Autodesk Fusion 360 part; units mm, degrees
(part 3 of 8)
  spline S11 degree 5 poles (2.5437, 23.8648) (2.5417, 23.8617) (2.5376, 23.8555) (2.5314, 23.8462) (2.5232, 23.8338) (2.5131, 23.8183) (2.503, 23.8028) (2.4929, 23.7874) (2.4829, 23.7719) (2.4729, 23.7565) (2.4629, 23.7411) (2.4531, 23.7257) (2.4432, 23.7103) (2.4334, 23.695) (2.4237, 23.6796) (2.414, 23.6643) (2.4044, 23.649) (2.3948, 23.6337) (2.3852, 23.6184) (2.3757, 23.6032) (2.3663, 23.588) (2.3569, 23.5727) (2.3475, 23.5575) (2.3382, 23.5424) (2.3289, 23.5272) (2.3197, 23.5121) (2.3105, 23.4969) (2.3014, 23.4818) (2.2923, 23.4668) (2.2833, 23.4517) (2.2743, 23.4367) (2.2654, 23.4216) (2.2565, 23.4066) (2.2477, 23.3917) (2.2389, 23.3767) (2.2302, 23.3618) (2.2215, 23.3468) (2.2128, 23.332) (2.2043, 23.3171) (2.1957, 23.3022) (2.1872, 23.2874) (2.1788, 23.2726) (2.1703, 23.2578) (2.162, 23.2431) (2.1537, 23.2283) (2.1454, 23.2136) (2.1372, 23.1989) (2.129, 23.1843) (2.1209, 23.1696) (2.1129, 23.155) (2.1048, 23.1404) (2.0969, 23.1259) (2.0889, 23.1113) (2.0811, 23.0968) (2.0732, 23.0823) (2.0654, 23.0679) (2.0577, 23.0535) (2.05, 23.039) (2.0424, 23.0247) (2.0348, 23.0103) (2.0272, 22.996) (2.0197, 22.9817) (2.0123, 22.9674) (2.0049, 22.9532) (1.9975, 22.939) (1.9902, 22.9248) (1.983, 22.9106) (1.9758, 22.8965) (1.9686, 22.8824) (1.9615, 22.8683) (1.9544, 22.8543) (1.9474, 22.8403) (1.9404, 22.8263) (1.9335, 22.8124) (1.9266, 22.7984) (1.9198, 22.7846) (1.913, 22.7707) (1.9063, 22.7569) (1.8996, 22.7431) (1.8929, 22.7293) (1.8863, 22.7156) (1.8798, 22.7019) (1.8733, 22.6883) (1.8668, 22.6747) (1.8604, 22.6611) (1.8541, 22.6475) (1.8478, 22.634) (1.8415, 22.6205) (1.8353, 22.6071) (1.8291, 22.5936) (1.823, 22.5803) (1.8169, 22.5669) (1.8109, 22.5536) (1.8049, 22.5403) (1.799, 22.5271) (1.7931, 22.5139) (1.7873, 22.5008) (1.7815, 22.4876) (1.7757, 22.4746) (1.77, 22.4615) (1.7644, 22.4485) (1.7588, 22.4356) (1.7532, 22.4226) (1.7477, 22.4097) (1.7423, 22.3969) (1.7368, 22.3841) (1.7315, 22.3713) (1.7261, 22.3586) (1.7209, 22.3459) (1.7156, 22.3333) (1.7105, 22.3207) (1.7053, 22.3082) (1.7002, 22.2956) (1.6952, 22.2832) (1.6902, 22.2708) (1.6853, 22.2584) (1.6803, 22.2461) (1.6755, 22.2338) (1.6707, 22.2215) (1.6659, 22.2093) (1.6612, 22.1972) (1.6565, 22.1851) (1.6519, 22.173) (1.6473, 22.161) (1.6428, 22.1491) (1.6383, 22.1372) (1.6339, 22.1253) (1.6295, 22.1135) (1.6251, 22.1017) (1.6208, 22.09) (1.6165, 22.0784) (1.6123, 22.0668) (1.6082, 22.0552) (1.604, 22.0437) (1.6, 22.0322) (1.5959, 22.0208) (1.592, 22.0095) (1.588, 21.9982) (1.5841, 21.987) (1.5803, 21.9758) (1.5765, 21.9646) (1.5727, 21.9536) (1.569, 21.9425) (1.5653, 21.9316) (1.5617, 21.9207) (1.5581, 21.9098) (1.5546, 21.899) (1.5511, 21.8883) (1.5476, 21.8776) (1.5442, 21.867) (1.5409, 21.8565) (1.5376, 21.846) (1.5343, 21.8356) (1.5311, 21.8252) (1.5279, 21.8149) (1.5247, 21.8047) (1.5216, 21.7945) (1.5186, 21.7844) (1.5156, 21.7743) (1.5126, 21.7644) (1.5097, 21.7544) (1.5068, 21.7446) (1.504, 21.7348) (1.5012, 21.7251) (1.4984, 21.7155) (1.4957, 21.7059) (1.4931, 21.6964) (1.4905, 21.687) (1.4879, 21.6776) (1.4853, 21.6683) (1.4828, 21.6591) (1.4804, 21.65) (1.478, 21.6409) (1.4756, 21.6319) (1.4733, 21.623) (1.471, 21.6142) (1.4688, 21.6054) (1.4666, 21.5967) (1.4644, 21.5881) (1.4623, 21.5796) (1.4602, 21.5711) (1.4582, 21.5628) (1.4562, 21.5545) (1.4542, 21.5463) (1.4523, 21.5382) (1.4504, 21.5302) (1.4486, 21.5222) (1.4468, 21.5144) (1.445, 21.5066) (1.4433, 21.4989) (1.4416, 21.4913) (1.44, 21.4838) (1.4384, 21.4764) (1.4368, 21.4691) (1.4353, 21.4619) (1.4338, 21.4548) (1.4324, 21.4478) (1.431, 21.4408) (1.4296, 21.434) (1.4283, 21.4273) (1.427, 21.4206) (1.4257, 21.4141) (1.4245, 21.4077) (1.4233, 21.4014) (1.4221, 21.3951) (1.421, 21.389) (1.4199, 21.383) (1.4189, 21.3771) (1.4179, 21.3714) (1.4169, 21.3657) (1.416, 21.3602) (1.4151, 21.3547) (1.4142, 21.3494) (1.4134, 21.3442) (1.4125, 21.3391) (1.4118, 21.3342) (1.411, 21.3293) (1.4103, 21.3246) (1.4096, 21.32) (1.409, 21.3156) (1.4084, 21.3113) (1.4078, 21.3071) (1.4072, 21.303) (1.4067, 21.2991) (1.4062, 21.2953) (1.4058, 21.2917) (1.4053, 21.2882) (1.4049, 21.2849) (1.4045, 21.2817) (1.4042, 21.2786) (1.4038, 21.2758) (1.4035, 21.273) (1.4033, 21.2705) (1.403, 21.2681) (1.4028, 21.2658) (1.4026, 21.2637) (1.4024, 21.2618) (1.4022, 21.2601) (1.4021, 21.2586) (1.402, 21.2572) (1.4019, 21.256) (1.4018, 21.2552) (1.4018, 21.2547) (1.4017, 21.2544) (1.4017, 21.2543) knots -1 -1 -1 -1 -1 -1 -0.99583333 -0.99166667 -0.9875 -0.98333333 -0.97916667 -0.975 -0.97083333 -0.96666667 -0.9625 -0.95833333 -0.95416667 -0.95 -0.94583333 -0.94166667 -0.9375 -0.93333333 -0.92916667 -0.925 -0.92083333 -0.91666667 -0.9125 -0.90833333 -0.90416667 -0.9 -0.89583333 -0.89166667 -0.8875 -0.88333333 -0.87916667 -0.875 -0.87083333 -0.86666667 -0.8625 -0.85833333 -0.85416667 -0.85 -0.84583333 -0.84166667 -0.8375 -0.83333333 -0.82916667 -0.825 -0.82083333 -0.81666667 -0.8125 -0.80833333 -0.80416667 -0.8 -0.79583333 -0.79166667 -0.7875 -0.78333333 -0.77916667 -0.775 -0.77083333 -0.76666667 -0.7625 -0.75833333 -0.75416667 -0.75 -0.74583333 -0.74166667 -0.7375 -0.73333333 -0.72916667 -0.725 -0.72083333 -0.71666667 -0.7125 -0.70833333 -0.70416667 -0.7 -0.69583333 -0.69166667 -0.6875 -0.68333333 -0.67916667 -0.675 -0.67083333 -0.66666667 -0.6625 -0.65833333 -0.65416667 -0.65 -0.64583333 -0.64166667 -0.6375 -0.63333333 -0.62916667 -0.625 -0.62083333 -0.61666667 -0.6125 -0.60833333 -0.60416667 -0.6 -0.59583333 -0.59166667 -0.5875 -0.58333333 -0.57916667 -0.575 -0.57083333 -0.56666667 -0.5625 -0.55833333 -0.55416667 -0.55 -0.54583333 -0.54166667 -0.5375 -0.53333333 -0.52916667 -0.525 -0.52083333 -0.51666667 -0.5125 -0.50833333 -0.50416667 -0.5 -0.49583333 -0.49166667 -0.4875 -0.48333333 -0.47916667 -0.475 -0.47083333 -0.46666667 -0.4625 -0.45833333 -0.45416667 -0.45 -0.44583333 -0.44166667 -0.4375 -0.43333333 -0.42916667 -0.425 -0.42083333 -0.41666667 -0.4125 -0.40833333 -0.40416667 -0.4 -0.39583333 -0.39166667 -0.3875 -0.38333333 -0.37916667 -0.375 -0.37083333 -0.36666667 -0.3625 -0.35833333 -0.35416667 -0.35 -0.34583333 -0.34166667 -0.3375 -0.33333333 -0.32916667 -0.325 -0.32083333 -0.31666667 -0.3125 -0.30833333 -0.30416667 -0.3 -0.29583333 -0.29166667 -0.2875 -0.28333333 -0.27916667 -0.275 -0.27083333 -0.26666667 -0.2625 -0.25833333 -0.25416667 -0.25 -0.24583333 -0.24166667 -0.2375 -0.23333333 -0.22916667 -0.225 -0.22083333 -0.21666667 -0.2125 -0.20833333 -0.20416667 -0.2 -0.19583333 -0.19166667 -0.1875 -0.18333333 -0.17916667 -0.175 -0.17083333 -0.16666667 -0.1625 -0.15833333 -0.15416667 -0.15 -0.14583333 -0.14166667 -0.1375 -0.13333333 -0.12916667 -0.125 -0.12083333 -0.11666667 -0.1125 -0.10833333 -0.10416667 -0.1 -0.09583333 -0.09166667 -0.0875 -0.08333333 -0.07916667 -0.075 -0.07083333 -0.06666667 -0.0625 -0.05833333 -0.05416667 -0.05 -0.04583333 -0.04166667 -0.0375 -0.03333333 -0.02916667 -0.025 -0.02083333 -0.01666667 -0.0125 -0.00833333 -0.00416667 0 0 0 0 0 0
  line L22 (1.4017, 21.2543) -> (1.4016, 21.2531)
  line L23 (1.4016, 21.2531) -> (1.2832, 19.4577)
  arc A12 (1.2832, 19.4577) -> (-1.2832, 19.4577) centre (0, 0) ccw
  line L24 (-1.2832, 19.4577) -> (-1.4016, 21.2531)
  line L25 (-1.4016, 21.2531) -> (-1.4017, 21.2543)
  spline S12 degree 5 poles (-1.4017, 21.2543) (-1.4017, 21.2544) (-1.4018, 21.2547) (-1.4018, 21.2552) (-1.4019, 21.256) (-1.402, 21.2572) (-1.4021, 21.2586) (-1.4022, 21.2601) (-1.4024, 21.2618) (-1.4026, 21.2637) (-1.4028, 21.2658) (-1.403, 21.2681) (-1.4033, 21.2705) (-1.4035, 21.273) (-1.4038, 21.2758) (-1.4042, 21.2786) (-1.4045, 21.2817) (-1.4049, 21.2849) (-1.4053, 21.2882) (-1.4058, 21.2917) (-1.4062, 21.2953) (-1.4067, 21.2991) (-1.4072, 21.303) (-1.4078, 21.3071) (-1.4084, 21.3113) (-1.409, 21.3156) (-1.4096, 21.32) (-1.4103, 21.3246) (-1.411, 21.3293) (-1.4118, 21.3342) (-1.4125, 21.3391) (-1.4134, 21.3442) (-1.4142, 21.3494) (-1.4151, 21.3547) (-1.416, 21.3602) (-1.4169, 21.3657) (-1.4179, 21.3714) (-1.4189, 21.3771) (-1.4199, 21.383) (-1.421, 21.389) (-1.4221, 21.3951) (-1.4233, 21.4014) (-1.4245, 21.4077) (-1.4257, 21.4141) (-1.427, 21.4206) (-1.4283, 21.4273) (-1.4296, 21.434) (-1.431, 21.4408) (-1.4324, 21.4478) (-1.4338, 21.4548) (-1.4353, 21.4619) (-1.4368, 21.4691) (-1.4384, 21.4764) (-1.44, 21.4838) (-1.4416, 21.4913) (-1.4433, 21.4989) (-1.445, 21.5066) (-1.4468, 21.5144) (-1.4486, 21.5222) (-1.4504, 21.5302) (-1.4523, 21.5382) (-1.4542, 21.5463) (-1.4562, 21.5545) (-1.4582, 21.5628) (-1.4602, 21.5711) (-1.4623, 21.5796) (-1.4644, 21.5881) (-1.4666, 21.5967) (-1.4688, 21.6054) (-1.471, 21.6142) (-1.4733, 21.623) (-1.4756, 21.6319) (-1.478, 21.6409) (-1.4804, 21.65) (-1.4828, 21.6591) (-1.4853, 21.6683) (-1.4879, 21.6776) (-1.4905, 21.687) (-1.4931, 21.6964) (-1.4957, 21.7059) (-1.4984, 21.7155) (-1.5012, 21.7251) (-1.504, 21.7348) (-1.5068, 21.7446) (-1.5097, 21.7544) (-1.5126, 21.7644) (-1.5156, 21.7743) (-1.5186, 21.7844) (-1.5216, 21.7945) (-1.5247, 21.8047) (-1.5279, 21.8149) (-1.5311, 21.8252) (-1.5343, 21.8356) (-1.5376, 21.846) (-1.5409, 21.8565) (-1.5442, 21.867) (-1.5476, 21.8776) (-1.5511, 21.8883) (-1.5546, 21.899) (-1.5581, 21.9098) (-1.5617, 21.9207) (-1.5653, 21.9316) (-1.569, 21.9425) (-1.5727, 21.9536) (-1.5765, 21.9646) (-1.5803, 21.9758) (-1.5841, 21.987) (-1.588, 21.9982) (-1.592, 22.0095) (-1.5959, 22.0208) (-1.6, 22.0322) (-1.604, 22.0437) (-1.6082, 22.0552) (-1.6123, 22.0668) (-1.6165, 22.0784) (-1.6208, 22.09) (-1.6251, 22.1017) (-1.6295, 22.1135) (-1.6339, 22.1253) (-1.6383, 22.1372) (-1.6428, 22.1491) (-1.6473, 22.161) (-1.6519, 22.173) (-1.6565, 22.1851) (-1.6612, 22.1972) (-1.6659, 22.2093) (-1.6707, 22.2215) (-1.6755, 22.2338) (-1.6803, 22.2461) (-1.6853, 22.2584) (-1.6902, 22.2708) (-1.6952, 22.2832) (-1.7002, 22.2956) (-1.7053, 22.3082) (-1.7105, 22.3207) (-1.7156, 22.3333) (-1.7209, 22.3459) (-1.7261, 22.3586) (-1.7315, 22.3713) (-1.7368, 22.3841) (-1.7423, 22.3969) (-1.7477, 22.4097) (-1.7532, 22.4226) (-1.7588, 22.4356) (-1.7644, 22.4485) (-1.77, 22.4615) (-1.7757, 22.4746) (-1.7815, 22.4876) (-1.7873, 22.5008) (-1.7931, 22.5139) (-1.799, 22.5271) (-1.8049, 22.5403) (-1.8109, 22.5536) (-1.8169, 22.5669) (-1.823, 22.5803) (-1.8291, 22.5936) (-1.8353, 22.6071) (-1.8415, 22.6205) (-1.8478, 22.634) (-1.8541, 22.6475) (-1.8604, 22.6611) (-1.8668, 22.6747) (-1.8733, 22.6883) (-1.8798, 22.7019) (-1.8863, 22.7156) (-1.8929, 22.7293) (-1.8996, 22.7431) (-1.9063, 22.7569) (-1.913, 22.7707) (-1.9198, 22.7846) (-1.9266, 22.7984) (-1.9335, 22.8124) (-1.9404, 22.8263) (-1.9474, 22.8403) (-1.9544, 22.8543) (-1.9615, 22.8683) (-1.9686, 22.8824) (-1.9758, 22.8965) (-1.983, 22.9106) (-1.9902, 22.9248) (-1.9975, 22.939) (-2.0049, 22.9532) (-2.0123, 22.9674) (-2.0197, 22.9817) (-2.0272, 22.996) (-2.0348, 23.0103) (-2.0424, 23.0247) (-2.05, 23.039) (-2.0577, 23.0535) (-2.0654, 23.0679) (-2.0732, 23.0823) (-2.0811, 23.0968) (-2.0889, 23.1113) (-2.0969, 23.1259) (-2.1048, 23.1404) (-2.1129, 23.155) (-2.1209, 23.1696) (-2.129, 23.1843) (-2.1372, 23.1989) (-2.1454, 23.2136) (-2.1537, 23.2283) (-2.162, 23.2431) (-2.1703, 23.2578) (-2.1788, 23.2726) (-2.1872, 23.2874) (-2.1957, 23.3022) (-2.2043, 23.3171) (-2.2128, 23.332) (-2.2215, 23.3468) (-2.2302, 23.3618) (-2.2389, 23.3767) (-2.2477, 23.3917) (-2.2565, 23.4066) (-2.2654, 23.4216) (-2.2743, 23.4367) (-2.2833, 23.4517) (-2.2923, 23.4668) (-2.3014, 23.4818) (-2.3105, 23.4969) (-2.3197, 23.5121) (-2.3289, 23.5272) (-2.3382, 23.5424) (-2.3475, 23.5575) (-2.3569, 23.5727) (-2.3663, 23.588) (-2.3757, 23.6032) (-2.3852, 23.6184) (-2.3948, 23.6337) (-2.4044, 23.649) (-2.414, 23.6643) (-2.4237, 23.6796) (-2.4334, 23.695) (-2.4432, 23.7103) (-2.4531, 23.7257) (-2.4629, 23.7411) (-2.4729, 23.7565) (-2.4829, 23.7719) (-2.4929, 23.7874) (-2.503, 23.8028) (-2.5131, 23.8183) (-2.5232, 23.8338) (-2.5314, 23.8462) (-2.5376, 23.8555) (-2.5417, 23.8617) (-2.5437, 23.8648) knots 0 0 0 0 0 0 0.00416667 0.00833333 0.0125 0.01666667 0.02083333 0.025 0.02916667 0.03333333 0.0375 0.04166667 0.04583333 0.05 0.05416667 0.05833333 0.0625 0.06666667 0.07083333 0.075 0.07916667 0.08333333 0.0875 0.09166667 0.09583333 0.1 0.10416667 0.10833333 0.1125 0.11666667 0.12083333 0.125 0.12916667 0.13333333 0.1375 0.14166667 0.14583333 0.15 0.15416667 0.15833333 0.1625 0.16666667 0.17083333 0.175 0.17916667 0.18333333 0.1875 0.19166667 0.19583333 0.2 0.20416667 0.20833333 0.2125 0.21666667 0.22083333 0.225 0.22916667 0.23333333 0.2375 0.24166667 0.24583333 0.25 0.25416667 0.25833333 0.2625 0.26666667 0.27083333 0.275 0.27916667 0.28333333 0.2875 0.29166667 0.29583333 0.3 0.30416667 0.30833333 0.3125 0.31666667 0.32083333 0.325 0.32916667 0.33333333 0.3375 0.34166667 0.34583333 0.35 0.35416667 0.35833333 0.3625 0.36666667 0.37083333 0.375 0.37916667 0.38333333 0.3875 0.39166667 0.39583333 0.4 0.40416667 0.40833333 0.4125 0.41666667 0.42083333 0.425 0.42916667 0.43333333 0.4375 0.44166667 0.44583333 0.45 0.45416667 0.45833333 0.4625 0.46666667 0.47083333 0.475 0.47916667 0.48333333 0.4875 0.49166667 0.49583333 0.5 0.50416667 0.50833333 0.5125 0.51666667 0.52083333 0.525 0.52916667 0.53333333 0.5375 0.54166667 0.54583333 0.55 0.55416667 0.55833333 0.5625 0.56666667 0.57083333 0.575 0.57916667 0.58333333 0.5875 0.59166667 0.59583333 0.6 0.60416667 0.60833333 0.6125 0.61666667 0.62083333 0.625 0.62916667 0.63333333 0.6375 0.64166667 0.64583333 0.65 0.65416667 0.65833333 0.6625 0.66666667 0.67083333 0.675 0.67916667 0.68333333 0.6875 0.69166667 0.69583333 0.7 0.70416667 0.70833333 0.7125 0.71666667 0.72083333 0.725 0.72916667 0.73333333 0.7375 0.74166667 0.74583333 0.75 0.75416667 0.75833333 0.7625 0.76666667 0.77083333 0.775 0.77916667 0.78333333 0.7875 0.79166667 0.79583333 0.8 0.80416667 0.80833333 0.8125 0.81666667 0.82083333 0.825 0.82916667 0.83333333 0.8375 0.84166667 0.84583333 0.85 0.85416667 0.85833333 0.8625 0.86666667 0.87083333 0.875 0.87916667 0.88333333 0.8875 0.89166667 0.89583333 0.9 0.90416667 0.90833333 0.9125 0.91666667 0.92083333 0.925 0.92916667 0.93333333 0.9375 0.94166667 0.94583333 0.95 0.95416667 0.95833333 0.9625 0.96666667 0.97083333 0.975 0.97916667 0.98333333 0.9875 0.99166667 0.99583333 1 1 1 1 1 1
  arc A13 (-2.5437, 23.8648) -> (-4.2828, 23.6148) centre (0, 0) ccw
  spline S13 degree 5 poles (-4.2828, 23.6148) (-4.2839, 23.6112) (-4.2861, 23.6041) (-4.2894, 23.5934) (-4.2937, 23.5792) (-4.2991, 23.5615) (-4.3045, 23.5438) (-4.3098, 23.5261) (-4.315, 23.5085) (-4.3203, 23.4909) (-4.3255, 23.4733) (-4.3306, 23.4558) (-4.3357, 23.4382) (-4.3408, 23.4207) (-4.3458, 23.4033) (-4.3508, 23.3858) (-4.3557, 23.3684) (-4.3606, 23.3511) (-4.3655, 23.3337) (-4.3703, 23.3164) (-4.3751, 23.2991) (-4.3798, 23.2819) (-4.3845, 23.2647) (-4.3892, 23.2475) (-4.3938, 23.2303) (-4.3984, 23.2132) (-4.4029, 23.1961) (-4.4074, 23.179) (-4.4119, 23.162) (-4.4163, 23.145) (-4.4206, 23.1281) (-4.425, 23.1111) (-4.4293, 23.0942) (-4.4335, 23.0774) (-4.4378, 23.0606) (-4.4419, 23.0438) (-4.4461, 23.027) (-4.4502, 23.0103) (-4.4542, 22.9936) (-4.4582, 22.9769) (-4.4622, 22.9603) (-4.4662, 22.9437) (-4.4701, 22.9272) (-4.4739, 22.9107) (-4.4777, 22.8942) (-4.4815, 22.8777) (-4.4853, 22.8613) (-4.489, 22.845) (-4.4926, 22.8286) (-4.4963, 22.8124) (-4.4998, 22.7961) (-4.5034, 22.7799) (-4.5069, 22.7637) (-4.5104, 22.7475) (-4.5138, 22.7314) (-4.5172, 22.7154) (-4.5206, 22.6993) (-4.5239, 22.6834) (-4.5272, 22.6674) (-4.5304, 22.6515) (-4.5336, 22.6356) (-4.5368, 22.6198) (-4.5399, 22.604) (-4.543, 22.5883) (-4.546, 22.5725) (-4.549, 22.5569) (-4.552, 22.5412) (-4.555, 22.5257) (-4.5579, 22.5101) (-4.5607, 22.4946) (-4.5636, 22.4792) (-4.5663, 22.4637) (-4.5691, 22.4484) (-4.5718, 22.433) (-4.5745, 22.4177) (-4.5771, 22.4025) (-4.5797, 22.3873) (-4.5823, 22.3721) (-4.5848, 22.357) (-4.5873, 22.3419) (-4.5898, 22.3269) (-4.5922, 22.3119) (-4.5946, 22.297) (-4.597, 22.2821) (-4.5993, 22.2673) (-4.6016, 22.2525) (-4.6038, 22.2377) (-4.606, 22.223) (-4.6082, 22.2084) (-4.6103, 22.1938) (-4.6124, 22.1792) (-4.6145, 22.1647) (-4.6165, 22.1502) (-4.6185, 22.1358) (-4.6205, 22.1214) (-4.6224, 22.1071) (-4.6243, 22.0929) (-4.6262, 22.0786) (-4.628, 22.0645) (-4.6298, 22.0503) (-4.6316, 22.0363) (-4.6333, 22.0223) (-4.635, 22.0083) (-4.6366, 21.9944) (-4.6383, 21.9805) (-4.6398, 21.9667) (-4.6414, 21.953) (-4.6429, 21.9392) (-4.6444, 21.9256) (-4.6459, 21.912) (-4.6473, 21.8985) (-4.6487, 21.885) (-4.65, 21.8715) (-4.6514, 21.8582) (-4.6527, 21.8448) (-4.6539, 21.8316) (-4.6552, 21.8183) (-4.6564, 21.8052) (-4.6575, 21.7921) (-4.6587, 21.779) (-4.6598, 21.7661) (-4.6608, 21.7531) (-4.6619, 21.7403) (-4.6629, 21.7275) (-4.6639, 21.7147) (-4.6648, 21.702) (-4.6657, 21.6894) (-4.6666, 21.6768) (-4.6675, 21.6643) (-4.6683, 21.6519) (-4.6691, 21.6395) (-4.6699, 21.6271) (-4.6706, 21.6149) (-4.6714, 21.6027) (-4.672, 21.5905) (-4.6727, 21.5785) (-4.6733, 21.5664) (-4.6739, 21.5545) (-4.6745, 21.5426) (-4.675, 21.5308) (-4.6756, 21.5191) (-4.676, 21.5074) (-4.6765, 21.4958) (-4.6769, 21.4842) (-4.6773, 21.4727) (-4.6777, 21.4613) (-4.6781, 21.45) (-4.6784, 21.4387) (-4.6787, 21.4275) (-4.679, 21.4163) (-4.6792, 21.4053) (-4.6795, 21.3943) (-4.6797, 21.3833) (-4.6798, 21.3725) (-4.68, 21.3617) (-4.6801, 21.351) (-4.6802, 21.3404) (-4.6803, 21.3298) (-4.6804, 21.3193) (-4.6804, 21.3089) (-4.6804, 21.2986) (-4.6804, 21.2883) (-4.6803, 21.2781) (-4.6803, 21.268) (-4.6802, 21.258) (-4.6801, 21.2481) (-4.68, 21.2382) (-4.6798, 21.2284) (-4.6797, 21.2187) (-4.6795, 21.2091) (-4.6793, 21.1995) (-4.6791, 21.1901) (-4.6788, 21.1807) (-4.6786, 21.1714) (-4.6783, 21.1622) (-4.678, 21.1531) (-4.6777, 21.144) (-4.6773, 21.1351) (-4.677, 21.1262) (-4.6766, 21.1174) (-4.6762, 21.1087) (-4.6758, 21.1002) (-4.6754, 21.0916) (-4.675, 21.0832) (-4.6745, 21.0749) (-4.6741, 21.0667) (-4.6736, 21.0585) (-4.6731, 21.0505) (-4.6726, 21.0426) (-4.6721, 21.0347) (-4.6716, 21.027) (-4.671, 21.0193) (-4.6705, 21.0117) (-4.6699, 21.0043) (-4.6693, 20.9969) (-4.6688, 20.9897) (-4.6682, 20.9825) (-4.6676, 20.9755) (-4.667, 20.9685) (-4.6664, 20.9617) (-4.6657, 20.955) (-4.6651, 20.9484) (-4.6645, 20.9418) (-4.6638, 20.9354) (-4.6632, 20.9292) (-4.6625, 20.923) (-4.6619, 20.9169) (-4.6612, 20.911) (-4.6606, 20.9051) (-4.6599, 20.8994) (-4.6592, 20.8938) (-4.6586, 20.8884) (-4.6579, 20.883) (-4.6573, 20.8778) (-4.6566, 20.8727) (-4.6559, 20.8677) (-4.6553, 20.8629) (-4.6546, 20.8582) (-4.654, 20.8536) (-4.6534, 20.8491) (-4.6527, 20.8448) (-4.6521, 20.8406) (-4.6515, 20.8366) (-4.6509, 20.8327) (-4.6503, 20.8289) (-4.6498, 20.8253) (-4.6492, 20.8218) (-4.6486, 20.8185) (-4.6481, 20.8153) (-4.6476, 20.8123) (-4.6471, 20.8095) (-4.6466, 20.8067) (-4.6462, 20.8042) (-4.6457, 20.8018) (-4.6453, 20.7996) (-4.6449, 20.7976) (-4.6446, 20.7957) (-4.6442, 20.794) (-4.6439, 20.7924) (-4.6437, 20.7911) (-4.6434, 20.7899) (-4.6433, 20.7892) (-4.6432, 20.7887) (-4.6431, 20.7884) (-4.6431, 20.7882) knots -1 -1 -1 -1 -1 -1 -0.99583333 -0.99166667 -0.9875 -0.98333333 -0.97916667 -0.975 -0.97083333 -0.96666667 -0.9625 -0.95833333 -0.95416667 -0.95 -0.94583333 -0.94166667 -0.9375 -0.93333333 -0.92916667 -0.925 -0.92083333 -0.91666667 -0.9125 -0.90833333 -0.90416667 -0.9 -0.89583333 -0.89166667 -0.8875 -0.88333333 -0.87916667 -0.875 -0.87083333 -0.86666667 -0.8625 -0.85833333 -0.85416667 -0.85 -0.84583333 -0.84166667 -0.8375 -0.83333333 -0.82916667 -0.825 -0.82083333 -0.81666667 -0.8125 -0.80833333 -0.80416667 -0.8 -0.79583333 -0.79166667 -0.7875 -0.78333333 -0.77916667 -0.775 -0.77083333 -0.76666667 -0.7625 -0.75833333 -0.75416667 -0.75 -0.74583333 -0.74166667 -0.7375 -0.73333333 -0.72916667 -0.725 -0.72083333 -0.71666667 -0.7125 -0.70833333 -0.70416667 -0.7 -0.69583333 -0.69166667 -0.6875 -0.68333333 -0.67916667 -0.675 -0.67083333 -0.66666667 -0.6625 -0.65833333 -0.65416667 -0.65 -0.64583333 -0.64166667 -0.6375 -0.63333333 -0.62916667 -0.625 -0.62083333 -0.61666667 -0.6125 -0.60833333 -0.60416667 -0.6 -0.59583333 -0.59166667 -0.5875 -0.58333333 -0.57916667 -0.575 -0.57083333 -0.56666667 -0.5625 -0.55833333 -0.55416667 -0.55 -0.54583333 -0.54166667 -0.5375 -0.53333333 -0.52916667 -0.525 -0.52083333 -0.51666667 -0.5125 -0.50833333 -0.50416667 -0.5 -0.49583333 -0.49166667 -0.4875 -0.48333333 -0.47916667 -0.475 -0.47083333 -0.46666667 -0.4625 -0.45833333 -0.45416667 -0.45 -0.44583333 -0.44166667 -0.4375 -0.43333333 -0.42916667 -0.425 -0.42083333 -0.41666667 -0.4125 -0.40833333 -0.40416667 -0.4 -0.39583333 -0.39166667 -0.3875 -0.38333333 -0.37916667 -0.375 -0.37083333 -0.36666667 -0.3625 -0.35833333 -0.35416667 -0.35 -0.34583333 -0.34166667 -0.3375 -0.33333333 -0.32916667 -0.325 -0.32083333 -0.31666667 -0.3125 -0.30833333 -0.30416667 -0.3 -0.29583333 -0.29166667 -0.2875 -0.28333333 -0.27916667 -0.275 -0.27083333 -0.26666667 -0.2625 -0.25833333 -0.25416667 -0.25 -0.24583333 -0.24166667 -0.2375 -0.23333333 -0.22916667 -0.225 -0.22083333 -0.21666667 -0.2125 -0.20833333 -0.20416667 -0.2 -0.19583333 -0.19166667 -0.1875 -0.18333333 -0.17916667 -0.175 -0.17083333 -0.16666667 -0.1625 -0.15833333 -0.15416667 -0.15 -0.14583333 -0.14166667 -0.1375 -0.13333333 -0.12916667 -0.125 -0.12083333 -0.11666667 -0.1125 -0.10833333 -0.10416667 -0.1 -0.09583333 -0.09166667 -0.0875 -0.08333333 -0.07916667 -0.075 -0.07083333 -0.06666667 -0.0625 -0.05833333 -0.05416667 -0.05 -0.04583333 -0.04166667 -0.0375 -0.03333333 -0.02916667 -0.025 -0.02083333 -0.01666667 -0.0125 -0.00833333 -0.00416667 0 0 0 0 0 0
  line L26 (-4.6431, 20.7882) -> (-4.6428, 20.7871)
  line L27 (-4.6428, 20.7871) -> (-4.2506, 19.0311)
  arc A14 (-4.2506, 19.0311) -> (-6.7131, 18.308) centre (0, 0) ccw
  line L28 (-6.7131, 18.308) -> (-7.3326, 19.9973)
  line L29 (-7.3326, 19.9973) -> (-7.333, 19.9984)
  spline S14 degree 5 poles (-7.333, 19.9984) (-7.333, 19.9985) (-7.3331, 19.9988) (-7.3333, 19.9993) (-7.3336, 20) (-7.334, 20.0011) (-7.3345, 20.0024) (-7.3351, 20.0039) (-7.3357, 20.0055) (-7.3364, 20.0073) (-7.3372, 20.0092) (-7.3381, 20.0113) (-7.339, 20.0135) (-7.34, 20.0159) (-7.3411, 20.0184) (-7.3422, 20.0211) (-7.3434, 20.0239) (-7.3446, 20.0269) (-7.346, 20.03) (-7.3474, 20.0332) (-7.3489, 20.0366) (-7.3504, 20.04) (-7.352, 20.0436) (-7.3537, 20.0474) (-7.3554, 20.0512) (-7.3572, 20.0552) (-7.3591, 20.0593) (-7.361, 20.0635) (-7.363, 20.0678) (-7.3651, 20.0722) (-7.3673, 20.0768) (-7.3695, 20.0814) (-7.3717, 20.0862) (-7.3741, 20.091) (-7.3765, 20.096) (-7.3789, 20.1011) (-7.3815, 20.1062) (-7.3841, 20.1115) (-7.3867, 20.1168) (-7.3895, 20.1223) (-7.3922, 20.1278) (-7.3951, 20.1335) (-7.398, 20.1392) (-7.401, 20.145) (-7.4041, 20.1509) (-7.4072, 20.1569) (-7.4103, 20.163) (-7.4136, 20.1692) (-7.4169, 20.1754) (-7.4203, 20.1818) (-7.4237, 20.1882) (-7.4272, 20.1947) (-7.4307, 20.2013) (-7.4344, 20.2079) (-7.4381, 20.2146) (-7.4418, 20.2214) (-7.4456, 20.2283) (-7.4495, 20.2353) (-7.4534, 20.2423) (-7.4574, 20.2494) (-7.4615, 20.2566) (-7.4656, 20.2638) (-7.4698, 20.2711) (-7.474, 20.2785) (-7.4784, 20.286) (-7.4827, 20.2935) (-7.4872, 20.3011) (-7.4917, 20.3087) (-7.4962, 20.3164) (-7.5008, 20.3242) (-7.5055, 20.332) (-7.5103, 20.3399) (-7.5151, 20.3479) (-7.5199, 20.3559) (-7.5249, 20.364) (-7.5298, 20.3721) (-7.5349, 20.3803) (-7.54, 20.3886) (-7.5452, 20.3969) (-7.5504, 20.4053) (-7.5557, 20.4137) (-7.5611, 20.4222) (-7.5665, 20.4307) (-7.5719, 20.4393) (-7.5775, 20.4479) (-7.5831, 20.4566) (-7.5887, 20.4653) (-7.5944, 20.4741) (-7.6002, 20.483) (-7.6061, 20.4919) (-7.612, 20.5008) (-7.6179, 20.5098) (-7.6239, 20.5188) (-7.63, 20.5279) (-7.6361, 20.537) (-7.6423, 20.5462) (-7.6486, 20.5554) (-7.6549, 20.5647) (-7.6613, 20.574) (-7.6677, 20.5834) (-7.6742, 20.5928) (-7.6807, 20.6022) (-7.6874, 20.6117) (-7.694, 20.6212) (-7.7008, 20.6308) (-7.7075, 20.6404) (-7.7144, 20.65) (-7.7213, 20.6597) (-7.7283, 20.6694) (-7.7353, 20.6792) (-7.7424, 20.689) (-7.7495, 20.6988) (-7.7567, 20.7087) (-7.7639, 20.7186) (-7.7713, 20.7286) (-7.7786, 20.7386) (-7.7861, 20.7486) (-7.7935, 20.7587) (-7.8011, 20.7688) (-7.8087, 20.7789) (-7.8164, 20.7891) (-7.8241, 20.7993) (-7.8319, 20.8095) (-7.8397, 20.8197) (-7.8476, 20.83) (-7.8555, 20.8404) (-7.8635, 20.8507) (-7.8716, 20.8611) (-7.8797, 20.8715) (-7.8879, 20.882) (-7.8961, 20.8925) (-7.9044, 20.903) (-7.9128, 20.9135) (-7.9212, 20.9241) (-7.9296, 20.9347) (-7.9382, 20.9453) (-7.9467, 20.9559) (-7.9554, 20.9666) (-7.9641, 20.9773) (-7.9728, 20.9881) (-7.9816, 20.9988) (-7.9905, 21.0096) (-7.9994, 21.0204) (-8.0084, 21.0312) (-8.0174, 21.0421) (-8.0265, 21.053) (-8.0356, 21.0639) (-8.0448, 21.0748) (-8.0541, 21.0858) (-8.0634, 21.0968) (-8.0727, 21.1078) (-8.0822, 21.1188) (-8.0916, 21.1298) (-8.1012, 21.1409) (-8.1108, 21.152) (-8.1204, 21.1631) (-8.1301, 21.1743) (-8.1398, 21.1854) (-8.1497, 21.1966) (-8.1595, 21.2078) (-8.1694, 21.219) (-8.1794, 21.2302) (-8.1894, 21.2415) (-8.1995, 21.2527) (-8.2097, 21.264) (-8.2198, 21.2754) (-8.2301, 21.2867) (-8.2404, 21.298) (-8.2508, 21.3094) (-8.2612, 21.3208) (-8.2716, 21.3322) (-8.2822, 21.3436) (-8.2927, 21.355) (-8.3034, 21.3665) (-8.314, 21.3779) (-8.3248, 21.3894) (-8.3356, 21.4009) (-8.3464, 21.4124) (-8.3573, 21.4239) (-8.3683, 21.4355) (-8.3793, 21.447) (-8.3903, 21.4586) (-8.4014, 21.4702) (-8.4126, 21.4817) (-8.4238, 21.4934) (-8.4351, 21.505) (-8.4464, 21.5166) (-8.4578, 21.5282) (-8.4693, 21.5399) (-8.4808, 21.5516) (-8.4923, 21.5633) (-8.5039, 21.5749) (-8.5155, 21.5867) (-8.5272, 21.5984) (-8.539, 21.6101) (-8.5508, 21.6218) (-8.5627, 21.6336) (-8.5746, 21.6453) (-8.5865, 21.6571) (-8.5986, 21.6689) (-8.6106, 21.6807) (-8.6227, 21.6925) (-8.6349, 21.7043) (-8.6471, 21.7161) (-8.6594, 21.7279) (-8.6718, 21.7397) (-8.6841, 21.7516) (-8.6966, 21.7634) (-8.7091, 21.7753) (-8.7216, 21.7871) (-8.7342, 21.799) (-8.7468, 21.8109) (-8.7595, 21.8228) (-8.7723, 21.8347) (-8.7851, 21.8465) (-8.7979, 21.8585) (-8.8108, 21.8704) (-8.8238, 21.8823) (-8.8368, 21.8942) (-8.8499, 21.9061) (-8.863, 21.9181) (-8.8761, 21.93) (-8.8893, 21.9419) (-8.9026, 21.9539) (-8.9159, 21.9658) (-8.9293, 21.9778) (-8.9427, 21.9897) (-8.9561, 22.0017) (-8.9697, 22.0137) (-8.9832, 22.0256) (-8.9968, 22.0376) (-9.0105, 22.0496) (-9.0242, 22.0616) (-9.038, 22.0735) (-9.0518, 22.0855) (-9.0657, 22.0975) (-9.0796, 22.1095) (-9.0936, 22.1215) (-9.1076, 22.1335) (-9.1217, 22.1455) (-9.1358, 22.1575) (-9.1471, 22.1671) (-9.1556, 22.1743) (-9.1613, 22.1791) (-9.1642, 22.1815) knots 0 0 0 0 0 0 0.00416667 0.00833333 0.0125 0.01666667 0.02083333 0.025 0.02916667 0.03333333 0.0375 0.04166667 0.04583333 0.05 0.05416667 0.05833333 0.0625 0.06666667 0.07083333 0.075 0.07916667 0.08333333 0.0875 0.09166667 0.09583333 0.1 0.10416667 0.10833333 0.1125 0.11666667 0.12083333 0.125 0.12916667 0.13333333 0.1375 0.14166667 0.14583333 0.15 0.15416667 0.15833333 0.1625 0.16666667 0.17083333 0.175 0.17916667 0.18333333 0.1875 0.19166667 0.19583333 0.2 0.20416667 0.20833333 0.2125 0.21666667 0.22083333 0.225 0.22916667 0.23333333 0.2375 0.24166667 0.24583333 0.25 0.25416667 0.25833333 0.2625 0.26666667 0.27083333 0.275 0.27916667 0.28333333 0.2875 0.29166667 0.29583333 0.3 0.30416667 0.30833333 0.3125 0.31666667 0.32083333 0.325 0.32916667 0.33333333 0.3375 0.34166667 0.34583333 0.35 0.35416667 0.35833333 0.3625 0.36666667 0.37083333 0.375 0.37916667 0.38333333 0.3875 0.39166667 0.39583333 0.4 0.40416667 0.40833333 0.4125 0.41666667 0.42083333 0.425 0.42916667 0.43333333 0.4375 0.44166667 0.44583333 0.45 0.45416667 0.45833333 0.4625 0.46666667 0.47083333 0.475 0.47916667 0.48333333 0.4875 0.49166667 0.49583333 0.5 0.50416667 0.50833333 0.5125 0.51666667 0.52083333 0.525 0.52916667 0.53333333 0.5375 0.54166667 0.54583333 0.55 0.55416667 0.55833333 0.5625 0.56666667 0.57083333 0.575 0.57916667 0.58333333 0.5875 0.59166667 0.59583333 0.6 0.60416667 0.60833333 0.6125 0.61666667 0.62083333 0.625 0.62916667 0.63333333 0.6375 0.64166667 0.64583333 0.65 0.65416667 0.65833333 0.6625 0.66666667 0.67083333 0.675 0.67916667 0.68333333 0.6875 0.69166667 0.69583333 0.7 0.70416667 0.70833333 0.7125 0.71666667 0.72083333 0.725 0.72916667 0.73333333 0.7375 0.74166667 0.74583333 0.75 0.75416667 0.75833333 0.7625 0.76666667 0.77083333 0.775 0.77916667 0.78333333 0.7875 0.79166667 0.79583333 0.8 0.80416667 0.80833333 0.8125 0.81666667 0.82083333 0.825 0.82916667 0.83333333 0.8375 0.84166667 0.84583333 0.85 0.85416667 0.85833333 0.8625 0.86666667 0.87083333 0.875 0.87916667 0.88333333 0.8875 0.89166667 0.89583333 0.9 0.90416667 0.90833333 0.9125 0.91666667 0.92083333 0.925 0.92916667 0.93333333 0.9375 0.94166667 0.94583333 0.95 0.95416667 0.95833333 0.9625 0.96666667 0.97083333 0.975 0.97916667 0.98333333 0.9875 0.99166667 0.99583333 1 1 1 1 1 1
  arc A15 (-9.1642, 22.1815) -> (-10.7624, 21.4516) centre (0, 0) ccw
  spline S15 degree 5 poles (-10.7624, 21.4516) (-10.7624, 21.4479) (-10.7625, 21.4404) (-10.7627, 21.4293) (-10.7628, 21.4144) (-10.763, 21.3959) (-10.7632, 21.3774) (-10.7633, 21.359) (-10.7634, 21.3406) (-10.7634, 21.3222) (-10.7634, 21.3039) (-10.7634, 21.2856) (-10.7634, 21.2673) (-10.7633, 21.2491) (-10.7632, 21.2309) (-10.7631, 21.2128) (-10.7629, 21.1947) (-10.7627, 21.1767) (-10.7625, 21.1586) (-10.7623, 21.1407) (-10.762, 21.1227) (-10.7617, 21.1049) (-10.7613, 21.087) (-10.761, 21.0692) (-10.7606, 21.0515) (-10.7601, 21.0337) (-10.7597, 21.0161) (-10.7592, 20.9984) (-10.7586, 20.9808) (-10.7581, 20.9633) (-10.7575, 20.9458) (-10.7569, 20.9283) (-10.7563, 20.9109) (-10.7556, 20.8935) (-10.7549, 20.8762) (-10.7542, 20.8589) (-10.7534, 20.8416) (-10.7526, 20.8244) (-10.7518, 20.8073) (-10.751, 20.7902) (-10.7501, 20.7731) (-10.7492, 20.7561) (-10.7483, 20.7391) (-10.7474, 20.7222) (-10.7464, 20.7053) (-10.7454, 20.6885) (-10.7444, 20.6717) (-10.7433, 20.6549) (-10.7422, 20.6382) (-10.7411, 20.6215) (-10.74, 20.6049) (-10.7388, 20.5884) (-10.7376, 20.5719) (-10.7364, 20.5554) (-10.7352, 20.539) (-10.7339, 20.5226) (-10.7326, 20.5063) (-10.7313, 20.49) (-10.7299, 20.4738) (-10.7285, 20.4576) (-10.7271, 20.4415) (-10.7257, 20.4254) (-10.7243, 20.4094) (-10.7228, 20.3934) (-10.7213, 20.3774) (-10.7198, 20.3616) (-10.7182, 20.3457) (-10.7167, 20.3299) (-10.7151, 20.3142) (-10.7135, 20.2985) (-10.7118, 20.2829) (-10.7101, 20.2673) (-10.7085, 20.2518) (-10.7067, 20.2363) (-10.705, 20.2209) (-10.7032, 20.2055) (-10.7015, 20.1902) (-10.6997, 20.1749) (-10.6978, 20.1597) (-10.696, 20.1445) (-10.6941, 20.1294) (-10.6922, 20.1144) (-10.6903, 20.0994) (-10.6884, 20.0844) (-10.6864, 20.0695) (-10.6844, 20.0547) (-10.6824, 20.0399) (-10.6804, 20.0252) (-10.6784, 20.0105) (-10.6763, 19.9959) (-10.6742, 19.9813) (-10.6721, 19.9668) (-10.67, 19.9524) (-10.6678, 19.938) (-10.6657, 19.9236) (-10.6635, 19.9093) (-10.6613, 19.8951) (-10.6591, 19.8809) (-10.6568, 19.8668) (-10.6546, 19.8528) (-10.6523, 19.8388) (-10.65, 19.8249) (-10.6477, 19.811) (-10.6453, 19.7972) (-10.643, 19.7834) (-10.6406, 19.7697) (-10.6383, 19.7561) (-10.6359, 19.7425) (-10.6334, 19.729) (-10.631, 19.7155) (-10.6286, 19.7021) (-10.6261, 19.6888) (-10.6236, 19.6755) (-10.6211, 19.6623) (-10.6186, 19.6492) (-10.6161, 19.6361) (-10.6135, 19.623) (-10.611, 19.6101) (-10.6084, 19.5972) (-10.6058, 19.5843) (-10.6032, 19.5716) (-10.6006, 19.5589) (-10.598, 19.5462) (-10.5953, 19.5337) (-10.5927, 19.5211) (-10.59, 19.5087) (-10.5874, 19.4963) (-10.5847, 19.484) (-10.582, 19.4718) (-10.5793, 19.4596) (-10.5765, 19.4475) (-10.5738, 19.4354) (-10.5711, 19.4234) (-10.5683, 19.4115) (-10.5655, 19.3997) (-10.5628, 19.3879) (-10.56, 19.3762) (-10.5572, 19.3646) (-10.5544, 19.353) (-10.5516, 19.3415) (-10.5488, 19.3301) (-10.546, 19.3188) (-10.5431, 19.3075) (-10.5403, 19.2963) (-10.5374, 19.2852) (-10.5346, 19.2741) (-10.5317, 19.2631) (-10.5289, 19.2522) (-10.526, 19.2414) (-10.5231, 19.2306) (-10.5202, 19.2199) (-10.5174, 19.2093) (-10.5145, 19.1988) (-10.5116, 19.1883) (-10.5087, 19.1779) (-10.5058, 19.1676) (-10.5029, 19.1574) (-10.5, 19.1472) (-10.4971, 19.1371) (-10.4942, 19.1271) (-10.4913, 19.1172) (-10.4884, 19.1074) (-10.4855, 19.0976) (-10.4826, 19.0879) (-10.4797, 19.0783) (-10.4768, 19.0688) (-10.4739, 19.0594) (-10.471, 19.05) (-10.4681, 19.0408) (-10.4652, 19.0316) (-10.4623, 19.0225) (-10.4595, 19.0135) (-10.4566, 19.0045) (-10.4537, 18.9957) (-10.4509, 18.9869) (-10.448, 18.9783) (-10.4452, 18.9697) (-10.4423, 18.9612) (-10.4395, 18.9528) (-10.4367, 18.9445) (-10.4338, 18.9362) (-10.431, 18.9281) (-10.4282, 18.9201) (-10.4254, 18.9121) (-10.4227, 18.9043) (-10.4199, 18.8965) (-10.4172, 18.8888) (-10.4144, 18.8812) (-10.4117, 18.8738) (-10.409, 18.8664) (-10.4063, 18.8591) (-10.4036, 18.8519) (-10.401, 18.8448) (-10.3983, 18.8378) (-10.3957, 18.8309) (-10.3931, 18.8241) (-10.3905, 18.8174) (-10.388, 18.8108) (-10.3854, 18.8043) (-10.3829, 18.7979) (-10.3804, 18.7917) (-10.378, 18.7855) (-10.3755, 18.7794) (-10.3731, 18.7735) (-10.3707, 18.7676) (-10.3683, 18.7619) (-10.366, 18.7562) (-10.3637, 18.7507) (-10.3614, 18.7453) (-10.3592, 18.74) (-10.357, 18.7348) (-10.3548, 18.7298) (-10.3527, 18.7248) (-10.3506, 18.72) (-10.3485, 18.7153) (-10.3465, 18.7107) (-10.3445, 18.7062) (-10.3425, 18.7019) (-10.3406, 18.6977) (-10.3388, 18.6936) (-10.3369, 18.6896) (-10.3352, 18.6858) (-10.3334, 18.6821) (-10.3318, 18.6785) (-10.3301, 18.675) (-10.3286, 18.6717) (-10.327, 18.6686) (-10.3256, 18.6655) (-10.3242, 18.6626) (-10.3228, 18.6599) (-10.3216, 18.6573) (-10.3203, 18.6548) (-10.3192, 18.6525) (-10.3181, 18.6503) (-10.3171, 18.6483) (-10.3161, 18.6465) (-10.3152, 18.6448) (-10.3144, 18.6432) (-10.3137, 18.6419) (-10.3131, 18.6406) (-10.3125, 18.6396) (-10.3122, 18.6389) (-10.3119, 18.6385) (-10.3118, 18.6382) (-10.3117, 18.6381) knots -1 -1 -1 -1 -1 -1 -0.99583333 -0.99166667 -0.9875 -0.98333333 -0.97916667 -0.975 -0.97083333 -0.96666667 -0.9625 -0.95833333 -0.95416667 -0.95 -0.94583333 -0.94166667 -0.9375 -0.93333333 -0.92916667 -0.925 -0.92083333 -0.91666667 -0.9125 -0.90833333 -0.90416667 -0.9 -0.89583333 -0.89166667 -0.8875 -0.88333333 -0.87916667 -0.875 -0.87083333 -0.86666667 -0.8625 -0.85833333 -0.85416667 -0.85 -0.84583333 -0.84166667 -0.8375 -0.83333333 -0.82916667 -0.825 -0.82083333 -0.81666667 -0.8125 -0.80833333 -0.80416667 -0.8 -0.79583333 -0.79166667 -0.7875 -0.78333333 -0.77916667 -0.775 -0.77083333 -0.76666667 -0.7625 -0.75833333 -0.75416667 -0.75 -0.74583333 -0.74166667 -0.7375 -0.73333333 -0.72916667 -0.725 -0.72083333 -0.71666667 -0.7125 -0.70833333 -0.70416667 -0.7 -0.69583333 -0.69166667 -0.6875 -0.68333333 -0.67916667 -0.675 -0.67083333 -0.66666667 -0.6625 -0.65833333 -0.65416667 -0.65 -0.64583333 -0.64166667 -0.6375 -0.63333333 -0.62916667 -0.625 -0.62083333 -0.61666667 -0.6125 -0.60833333 -0.60416667 -0.6 -0.59583333 -0.59166667 -0.5875 -0.58333333 -0.57916667 -0.575 -0.57083333 -0.56666667 -0.5625 -0.55833333 -0.55416667 -0.55 -0.54583333 -0.54166667 -0.5375 -0.53333333 -0.52916667 -0.525 -0.52083333 -0.51666667 -0.5125 -0.50833333 -0.50416667 -0.5 -0.49583333 -0.49166667 -0.4875 -0.48333333 -0.47916667 -0.475 -0.47083333 -0.46666667 -0.4625 -0.45833333 -0.45416667 -0.45 -0.44583333 -0.44166667 -0.4375 -0.43333333 -0.42916667 -0.425 -0.42083333 -0.41666667 -0.4125 -0.40833333 -0.40416667 -0.4 -0.39583333 -0.39166667 -0.3875 -0.38333333 -0.37916667 -0.375 -0.37083333 -0.36666667 -0.3625 -0.35833333 -0.35416667 -0.35 -0.34583333 -0.34166667 -0.3375 -0.33333333 -0.32916667 -0.325 -0.32083333 -0.31666667 -0.3125 -0.30833333 -0.30416667 -0.3 -0.29583333 -0.29166667 -0.2875 -0.28333333 -0.27916667 -0.275 -0.27083333 -0.26666667 -0.2625 -0.25833333 -0.25416667 -0.25 -0.24583333 -0.24166667 -0.2375 -0.23333333 -0.22916667 -0.225 -0.22083333 -0.21666667 -0.2125 -0.20833333 -0.20416667 -0.2 -0.19583333 -0.19166667 -0.1875 -0.18333333 -0.17916667 -0.175 -0.17083333 -0.16666667 -0.1625 -0.15833333 -0.15416667 -0.15 -0.14583333 -0.14166667 -0.1375 -0.13333333 -0.12916667 -0.125 -0.12083333 -0.11666667 -0.1125 -0.10833333 -0.10416667 -0.1 -0.09583333 -0.09166667 -0.0875 -0.08333333 -0.07916667 -0.075 -0.07083333 -0.06666667 -0.0625 -0.05833333 -0.05416667 -0.05 -0.04583333 -0.04166667 -0.0375 -0.03333333 -0.02916667 -0.025 -0.02083333 -0.01666667 -0.0125 -0.00833333 -0.00416667 0 0 0 0 0 0
  line L30 (-10.3117, 18.6381) -> (-10.3111, 18.637)
  line L31 (-10.3111, 18.637) -> (-9.4401, 17.0627)
  arc A16 (-9.4401, 17.0627) -> (-11.5992, 15.6751) centre (0, 0) ccw
  line L32 (-11.5992, 15.6751) -> (-12.6694, 17.1214)
  line L33 (-12.6694, 17.1214) -> (-12.6701, 17.1224)
  spline S16 degree 5 poles (-12.6701, 17.1224) (-12.6702, 17.1225) (-12.6704, 17.1228) (-12.6707, 17.1232) (-12.6712, 17.1238) (-12.6719, 17.1247) (-12.6728, 17.1258) (-12.6737, 17.127) (-12.6748, 17.1284) (-12.676, 17.1299) (-12.6773, 17.1315) (-12.6787, 17.1333) (-12.6802, 17.1352) (-12.6818, 17.1372) (-12.6835, 17.1393) (-12.6854, 17.1416) (-12.6873, 17.1439) (-12.6894, 17.1464) (-12.6915, 17.149) (-12.6938, 17.1517) (-12.6961, 17.1545) (-12.6986, 17.1574) (-12.7011, 17.1604) (-12.7038, 17.1635) (-12.7065, 17.1667) (-12.7094, 17.17) (-12.7124, 17.1734) (-12.7154, 17.1769) (-12.7185, 17.1805) (-12.7218, 17.1842) (-12.7251, 17.1879) (-12.7285, 17.1918) (-12.732, 17.1957) (-12.7357, 17.1997) (-12.7394, 17.2038) (-12.7432, 17.2079) (-12.747, 17.2122) (-12.751, 17.2165) (-12.7551, 17.2209) (-12.7592, 17.2253) (-12.7635, 17.2299) (-12.7678, 17.2345) (-12.7722, 17.2392) (-12.7767, 17.2439) (-12.7813, 17.2487) (-12.786, 17.2536) (-12.7908, 17.2585) (-12.7956, 17.2635) (-12.8005, 17.2686) (-12.8055, 17.2737) (-12.8106, 17.2789) (-12.8158, 17.2842) (-12.8211, 17.2895) (-12.8264, 17.2948) (-12.8319, 17.3003) (-12.8374, 17.3057) (-12.843, 17.3113) (-12.8487, 17.3168) (-12.8544, 17.3225) (-12.8603, 17.3282) (-12.8662, 17.3339) (-12.8722, 17.3397) (-12.8783, 17.3455) (-12.8844, 17.3514) (-12.8906, 17.3574) (-12.897, 17.3633) (-12.9033, 17.3694) (-12.9098, 17.3754) (-12.9164, 17.3815) (-12.923, 17.3877) (-12.9297, 17.3939) (-12.9365, 17.4001) (-12.9433, 17.4064) (-12.9502, 17.4127) (-12.9572, 17.4191) (-12.9643, 17.4255) (-12.9715, 17.432) (-12.9787, 17.4384) (-12.986, 17.445) (-12.9934, 17.4515) (-13.0008, 17.4581) (-13.0084, 17.4647) (-13.016, 17.4714) (-13.0236, 17.4781) (-13.0314, 17.4848) (-13.0392, 17.4916) (-13.0471, 17.4984) (-13.055, 17.5052) (-13.0631, 17.512) (-13.0712, 17.5189) (-13.0794, 17.5258) (-13.0876, 17.5328) (-13.0959, 17.5398) (-13.1043, 17.5468) (-13.1128, 17.5538) (-13.1213, 17.5609) (-13.1299, 17.5679) (-13.1386, 17.575) (-13.1473, 17.5822) (-13.1561, 17.5893) (-13.165, 17.5965) (-13.1739, 17.6037) (-13.1829, 17.611) (-13.192, 17.6182) (-13.2012, 17.6255) (-13.2104, 17.6328) (-13.2197, 17.6402) (-13.229, 17.6475) (-13.2385, 17.6549) (-13.2479, 17.6623) (-13.2575, 17.6697) (-13.2671, 17.6771) (-13.2768, 17.6846) (-13.2866, 17.692) (-13.2964, 17.6995) (-13.3063, 17.707) (-13.3162, 17.7146) (-13.3262, 17.7221) (-13.3363, 17.7297) (-13.3465, 17.7372) (-13.3567, 17.7448) (-13.367, 17.7524) (-13.3773, 17.7601) (-13.3877, 17.7677) (-13.3982, 17.7754) (-13.4087, 17.783) (-13.4193, 17.7907) (-13.43, 17.7984) (-13.4407, 17.8061) (-13.4515, 17.8138) (-13.4624, 17.8216) (-13.4733, 17.8293) (-13.4843, 17.8371) (-13.4953, 17.8448) (-13.5064, 17.8526) (-13.5176, 17.8604) (-13.5288, 17.8682) (-13.5401, 17.876) (-13.5515, 17.8839) (-13.5629, 17.8917) (-13.5744, 17.8995) (-13.5859, 17.9074) (-13.5975, 17.9152) (-13.6092, 17.9231) (-13.6209, 17.931) (-13.6327, 17.9389) (-13.6445, 17.9468) (-13.6564, 17.9547) (-13.6684, 17.9626) (-13.6804, 17.9705) (-13.6925, 17.9784) (-13.7046, 17.9863) (-13.7168, 17.9943) (-13.7291, 18.0022) (-13.7414, 18.0101) (-13.7538, 18.0181) (-13.7662, 18.026) (-13.7787, 18.034) (-13.7913, 18.0419) (-13.8039, 18.0499) (-13.8166, 18.0579) (-13.8293, 18.0658) (-13.8421, 18.0738) (-13.855, 18.0818) (-13.8679, 18.0898) (-13.8808, 18.0978) (-13.8939, 18.1057) (-13.907, 18.1137) (-13.9201, 18.1217) (-13.9333, 18.1297) (-13.9465, 18.1377) (-13.9598, 18.1457) (-13.9732, 18.1536) (-13.9866, 18.1616) (-14.0001, 18.1696) (-14.0137, 18.1776) (-14.0272, 18.1856) (-14.0409, 18.1936) (-14.0546, 18.2016) (-14.0684, 18.2096) (-14.0822, 18.2175) (-14.096, 18.2255) (-14.11, 18.2335) (-14.124, 18.2415) (-14.138, 18.2494) (-14.1521, 18.2574) (-14.1662, 18.2654) (-14.1804, 18.2734) (-14.1947, 18.2813) (-14.209, 18.2893) (-14.2234, 18.2972) (-14.2378, 18.3052) (-14.2523, 18.3131) (-14.2668, 18.3211) (-14.2814, 18.329) (-14.296, 18.337) (-14.3107, 18.3449) (-14.3254, 18.3528) (-14.3402, 18.3607) (-14.3551, 18.3686) (-14.37, 18.3766) (-14.3849, 18.3845) (-14.3999, 18.3924) (-14.415, 18.4002) (-14.4301, 18.4081) (-14.4453, 18.416) (-14.4605, 18.4239) (-14.4758, 18.4317) (-14.4911, 18.4396) (-14.5065, 18.4474) (-14.5219, 18.4553) (-14.5374, 18.4631) (-14.5529, 18.4709) (-14.5685, 18.4788) (-14.5841, 18.4866) (-14.5998, 18.4944) (-14.6155, 18.5022) (-14.6313, 18.5099) (-14.6472, 18.5177) (-14.663, 18.5255) (-14.679, 18.5332) (-14.695, 18.541) (-14.711, 18.5487) (-14.7271, 18.5564) (-14.7432, 18.5642) (-14.7594, 18.5719) (-14.7757, 18.5796) (-14.792, 18.5872) (-14.8083, 18.5949) (-14.8247, 18.6026) (-14.8411, 18.6102) (-14.8576, 18.6179) (-14.8741, 18.6255) (-14.8907, 18.6331) (-14.9074, 18.6407) (-14.9241, 18.6483) (-14.9408, 18.6559) (-14.9576, 18.6635) (-14.9744, 18.671) (-14.9913, 18.6786) (-15.0082, 18.6861) (-15.0218, 18.6921) (-15.032, 18.6966) (-15.0388, 18.6996) (-15.0422, 18.7011) knots 0 0 0 0 0 0 0.00416667 0.00833333 0.0125 0.01666667 0.02083333 0.025 0.02916667 0.03333333 0.0375 0.04166667 0.04583333 0.05 0.05416667 0.05833333 0.0625 0.06666667 0.07083333 0.075 0.07916667 0.08333333 0.0875 0.09166667 0.09583333 0.1 0.10416667 0.10833333 0.1125 0.11666667 0.12083333 0.125 0.12916667 0.13333333 0.1375 0.14166667 0.14583333 0.15 0.15416667 0.15833333 0.1625 0.16666667 0.17083333 0.175 0.17916667 0.18333333 0.1875 0.19166667 0.19583333 0.2 0.20416667 0.20833333 0.2125 0.21666667 0.22083333 0.225 0.22916667 0.23333333 0.2375 0.24166667 0.24583333 0.25 0.25416667 0.25833333 0.2625 0.26666667 0.27083333 0.275 0.27916667 0.28333333 0.2875 0.29166667 0.29583333 0.3 0.30416667 0.30833333 0.3125 0.31666667 0.32083333 0.325 0.32916667 0.33333333 0.3375 0.34166667 0.34583333 0.35 0.35416667 0.35833333 0.3625 0.36666667 0.37083333 0.375 0.37916667 0.38333333 0.3875 0.39166667 0.39583333 0.4 0.40416667 0.40833333 0.4125 0.41666667 0.42083333 0.425 0.42916667 0.43333333 0.4375 0.44166667 0.44583333 0.45 0.45416667 0.45833333 0.4625 0.46666667 0.47083333 0.475 0.47916667 0.48333333 0.4875 0.49166667 0.49583333 0.5 0.50416667 0.50833333 0.5125 0.51666667 0.52083333 0.525 0.52916667 0.53333333 0.5375 0.54166667 0.54583333 0.55 0.55416667 0.55833333 0.5625 0.56666667 0.57083333 0.575 0.57916667 0.58333333 0.5875 0.59166667 0.59583333 0.6 0.60416667 0.60833333 0.6125 0.61666667 0.62083333 0.625 0.62916667 0.63333333 0.6375 0.64166667 0.64583333 0.65 0.65416667 0.65833333 0.6625 0.66666667 0.67083333 0.675 0.67916667 0.68333333 0.6875 0.69166667 0.69583333 0.7 0.70416667 0.70833333 0.7125 0.71666667 0.72083333 0.725 0.72916667 0.73333333 0.7375 0.74166667 0.74583333 0.75 0.75416667 0.75833333 0.7625 0.76666667 0.77083333 0.775 0.77916667 0.78333333 0.7875 0.79166667 0.79583333 0.8 0.80416667 0.80833333 0.8125 0.81666667 0.82083333 0.825 0.82916667 0.83333333 0.8375 0.84166667 0.84583333 0.85 0.85416667 0.85833333 0.8625 0.86666667 0.87083333 0.875 0.87916667 0.88333333 0.8875 0.89166667 0.89583333 0.9 0.90416667 0.90833333 0.9125 0.91666667 0.92083333 0.925 0.92916667 0.93333333 0.9375 0.94166667 0.94583333 0.95 0.95416667 0.95833333 0.9625 0.96666667 0.97083333 0.975 0.97916667 0.98333333 0.9875 0.99166667 0.99583333 1 1 1 1 1 1
  arc A17 (-15.0422, 18.7011) -> (-16.37, 17.5506) centre (0, 0) ccw